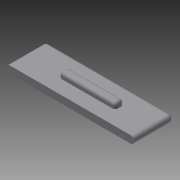
# Autodesk Inventor part: 160409 T-RH-P Box cap R23p
Saved by Autodesk Inventor 2015 (Build 190159000, 159)
## iProperties
Created: 2015-12-10
Part Number: 160409 T-RH-P Box cap R23p
Material: Generico
Document SubType Name: Modeling
Designer: piscian
Density: 1 g/cm^3
Appearance: Default
Author: piscian
Autodesk Inventor part; units mm, degrees
ref_plane "YZ Plane" through (0, 0, 0) normal (1, 0, 0) x (0, 1, 0)
ref_plane "XZ Plane" through (0, 0, 0) normal (0, 1, 0) x (-1, 0, 0)
ref_plane "XY Plane" through (0, 0, 0) normal (0, 0, 1) x (1, 0, 0)
sketch "Schizzo1" plane through (0, 0, 0) normal (0, 0, 1) x (1, 0, 0)
  line L0 (0, 0) -> (22.7, 0)
  line L1 (22.7, 0) -> (22.7, 7)
  line L2 (22.7, 7) -> (0, 7)
  line L3 (0, 7) -> (0, 0)
  dimension "d0" = 22.7
  dimension "d2" = 7
  constraints: 8 end point, 2 parallel, 1 horizontal, 1 perpendicular
  measures "d0" distance of L1.end L2.end
  measures "d2" distance of L2.end L0.start
extrude "Estrusione1" add sketch "Schizzo1" along normal blind 1.3
sketch "Sketch2" plane through (0, 0, 1.3) normal (0, 0, 1) x (1, 0, 0)
  line L0 (6.85, 4) -> (16.85, 4)
  line L1 (16.85, 4) -> (16.85, 2.5)
  line L2 (16.85, 2.5) -> (6.85, 2.5)
  line L3 (6.85, 2.5) -> (6.85, 4)
  line L4 (0, 7) -> (0, 0) projected
  line L5 (0, 0) -> (22.7, 0) projected
  point P0 (0, 6.5)
  dimension "d6" = 10
  dimension "d7" = 1.5
  dimension "d8" = 6.85
  dimension "d9" = 2.5
  constraints: 8 end point, 2 parallel, 1 horizontal, 1 perpendicular
  measures "d6" distance of L0.start L0.end
  measures "d7" distance of L2.end L0.start
  measures "d8" distance between parallel lines of L3 L4
  measures "d9" distance between parallel lines of L2 L5
extrude "Handle" add sketch "Sketch2" along normal blind 1
fillet "Fillet2" radius 0.5 8 edges at (16.85, 4, 1.8) (16.85, 2.5, 1.8) (6.85, 4, 1.8) (6.85, 2.5, 1.8) (11.85, 2.5, 2.3) (16.85, 3.25, 2.3) (6.85, 3.25, 2.3) (11.85, 4, 2.3)
fillet "Fillet3" radius 0.6 8 edges at (0, 7, 0.65) (22.7, 7, 0.65) (0, 3.5, 1.3) (0, 3.5, 0) (22.7, 3.5, 1.3) (22.7, 3.5, 0) (11.35, 7, 1.3) (11.35, 7, 0)
